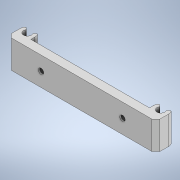
# Autodesk Inventor part: switch_mount
Saved by Autodesk Inventor 2020 (Build 240168000, 168)
## iProperties
Created: 2020-06-05
Part Number: switch_mount
Material: Generic
Document SubType Name: Modeling
Designer: suhren
Density: 1 g/cm^3
Appearance: Default
Author: suhren
Autodesk Inventor part; units mm, degrees
ref_plane "YZ Plane" through (0, 0, 0) normal (1, 0, 0) x (0, 1, 0)
ref_plane "XZ Plane" through (0, 0, 0) normal (0, 1, 0) x (-1, 0, 0)
ref_plane "XY Plane" through (0, 0, 0) normal (0, 0, 1) x (1, 0, 0)
sketch "Sketch1" plane through (0, 0, 0) normal (0, 1, 0) x (-1, 0, 0)
  line L0 (52.8, -3) -> (-52.8, -3) construction
  line L1 (-52.8, -3) -> (-52.8, 3)
  line L2 (-52.8, 3) -> (52.8, 3) construction
  line L3 (52.8, 3) -> (52.8, -3)
  circle A0 centre (47.5, -5.8) radius 2.8 construction
  circle A1 centre (-47.5, -5.8) radius 2.8 construction
  line L4 (50.3, -5.8) -> (50.3, -3) construction
  line L5 (44.7, -5.8) -> (44.7, -3) construction
  circle A2 centre (47.5, -5.8) radius 5.3 construction
  line L6 (52.8, -5.8) -> (52.8, -3)
  line L7 (42.2, -5.8) -> (42.2, -3)
  arc A3 (51.7589, -8.9546) -> (52.8, -5.8) centre (47.5, -5.8) ccw
  arc A4 (42.2, -5.8) -> (43.2411, -8.9546) centre (47.5, -5.8) ccw
  circle A5 centre (-47.5, -5.8) radius 5.3 construction
  line L8 (0, -3) -> (0, 3) construction
  line L9 (47.5, -5.8) -> (47.5, -3) construction
  line L10 (-47.5, -5.8) -> (-47.5, -3) construction
  line L11 (-42.2, -5.8) -> (-42.2, -3)
  line L12 (-52.8, -5.8) -> (-52.8, -3)
  arc A6 (-43.2411, -8.9546) -> (-42.2, -5.8) centre (-47.5, -5.8) ccw
  arc A7 (-52.8, -5.8) -> (-51.7589, -8.9546) centre (-47.5, -5.8) ccw
  line L13 (42.2, -3) -> (-42.2, -3)
  arc A8 (49.75, -7.4666) -> (45.25, -7.4666) centre (47.5, -5.8) ccw
  line L14 (49.75, -7.4666) -> (51.7589, -8.9546)
  line L15 (45.25, -7.4666) -> (43.2411, -8.9546)
  arc A9 (-45.25, -7.4666) -> (-49.75, -7.4666) centre (-47.5, -5.8) ccw
  line L16 (-45.25, -7.4666) -> (-43.2411, -8.9546)
  line L17 (-49.75, -7.4666) -> (-51.7589, -8.9546)
  line L18 (50, 3) -> (-50, 3)
  line L19 (-50, 3) -> (-52.8, 0.2)
  line L20 (50, 3) -> (52.8, 0.2)
  point P0 (0, 0)
  point P1 (0, 0)
  point P2 (47.5, -3)
  point P3 (-53.25, -3)
  dimension "d0" = 95
  dimension "d1" = 2.5
  dimension "d4" = 6
  dimension "d5" = 6
  dimension "d20" = 5.6
  dimension "d21" = 4.5
  dimension "d22" = 100
  constraints: 40 end point, 25 point on circle, 9 centre point, 8 vertical, 7 horizontal alignment, 5 coincident, 5 point on line, 5 tangent, 4 concentric, 3 perpendicular, 2 line through centre, 2 midpoint, 2 parallel, 1 equal radius, 1 horizontal, 1 symmetric about line, 1 vertical alignment, 20 other
  measures "d0" distance of point (-47.5, -5.8) A0.centre
  measures "d1" distance between parallel lines of L6 L4
  measures "d4" vertical distance of L2.end point (47.5, -3)
  measures "d5" distance of L3.end L2.end
  measures "d20" diameter of A0
  measures "d21" distance of L15.start L14.start
  measures "d22" distance of L18.start L18.end
extrude "Extrusion1" add sketch "Sketch1" along normal blind 20
fillet "Fillet1" radius 0.5 8 edges at (45.25, 10, -7.4666) (43.2411, 10, -8.9546) (51.7589, 10, -8.9546) (49.75, 10, -7.4666) (-51.7589, 10, -8.9546) (-49.75, 10, -7.4666) (-43.2411, 10, -8.9546) (-45.25, 10, -7.4666)
sketch "Sketch2" plane through (42.2, 0, -3) normal (0, 0, -1) x (-1, 0, 0)
  line L0 (0, 0) -> (84.4, 0) construction
  line L1 (0, 20) -> (84.4, 20) construction
  line L2 (42.2, 20) -> (42.2, 0) construction
  line L3 (13.2, 10) -> (71.2, 10) construction
  line L4 (9.7, 12.0207) -> (13.2, 14.0415)
  line L5 (13.2, 14.0415) -> (16.7, 12.0207)
  line L6 (16.7, 12.0207) -> (16.7, 7.9793)
  line L7 (16.7, 7.9793) -> (13.2, 5.9585)
  line L8 (13.2, 5.9585) -> (9.7, 7.9793)
  line L9 (9.7, 7.9793) -> (9.7, 12.0207)
  line L10 (74.7, 12.0207) -> (74.7, 7.9793)
  line L11 (74.7, 7.9793) -> (71.2, 5.9585)
  line L12 (71.2, 5.9585) -> (67.7, 7.9793)
  line L13 (67.7, 7.9793) -> (67.7, 12.0207)
  line L14 (67.7, 12.0207) -> (71.2, 14.0415)
  line L15 (71.2, 14.0415) -> (74.7, 12.0207)
  point P0 (42.2, 10)
  point P1 (42.2, 10)
  dimension "d9" = 58
  dimension "d10" = 7
  constraints: 28 end point, 4 coincident, 3 midpoint, 3 vertical, 1 horizontal, 1 parallel, 26 other
  measures "d9" distance of L3.start L3.end
  measures "d10" distance between parallel lines of L6 L9
extrude "Extrusion2" cut sketch "Sketch2" against normal blind 5
hole "Hole1" at (29, 10, -3) at (-29, 10, -3) direction (0, 0, 1) diameter 3.9 end through all
body "Solid1"
